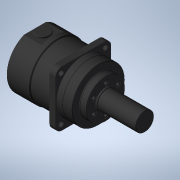
# Autodesk Inventor part: HPG-32A-33-J2NELA(400)
Saved by Autodesk Inventor 2021 (Build 250183000, 183)
## iProperties
Created: 2025-02-20
Part Number: HPG-32A-33-J2NELA(400)
Material: Generic
Catalog Web Link: www.cadenas.de
Description: HPG-32A-
Vendor: HARMONIC
Document SubType Name: Modeling
Designer: psAdmin
Manufacturer: HARMONIC
Mass: 1664.6 g
Surface Area: 1195.64 cm^2
Volume: 1664.6 cm^3
Density: 1 g/cm^3
Appearance: PSOLRGB-175-175-175
Category: PARTsolutions
Company: HARMONIC
Title: HPG-32A-33-J2NELA
Author: Cadenas PARTsolutions
PSOL_IDENT_0: {$CADENAS_DATA/23d-libs/harmonicdrive/data/hpg_series/selection_for_order_number/3d/shaft_output_no_
PSOL_IDENT_1: key_way/hpg_32a_j2.prj},182 {VTYP=3D},{NB=HPG-32A-33-J2NELA(400)},{LINA=HPG-32A-33-J2NELA},{NN=HPG-3
PSOL_IDENT_2: 2A},{DATE=16.11.2023 08:26:27},{GEOMDATE=09.08.2021 10:42:12},{VERSION=},{LINEID=4630},{WBVAR=},{WBN
PSOL_IDENT_3: UMERIC=}  {NB=HPG-32A-33-J2NELA(400)},{LINA=HPG-32A-33-J2NELA},{KT=DUMMY},{CNSORDERNO=HPG-32A-33-J2N
PSOL_IDENT_4: ELA},{R=33},{MC=400},{FN=NELA},{CNSORDERNO26=J2},{CNSORDERNO2=HPG-32A-33-J_NELA},{SB=0},{VERX=1}
NB: HPG-32A-33-J2NELA(400)
NN: HPG-32A
NBSYN: $CNSORDERNO.($MC.)
LINA: HPG-32A-33-J2NELA
CATALOG: Harmonic Drive
CNSORDERNO: HPG-32A-33-J2NELA
R: 33
MC: 400
FN: NELA
VERX: 1
SUPPLIER: HARMONIC
ARTICLENO: HPG-32A-33-J2NELA(400)
BOMINFO: HPG-32A-33-J2NELA
CREATOR: CADENAS GmbH
Autodesk Inventor part; units mm, degrees
ref_plane "YZ Plane" through (0, 0, 0) normal (1, 0, 0) x (0, 1, 0)
ref_plane "XZ Plane" through (0, 0, 0) normal (0, 1, 0) x (-1, 0, 0)
ref_plane "XY Plane" through (0, 0, 0) normal (0, 0, 1) x (1, 0, 0)
sketch "Sketch_1" plane through (0, 0, 0) normal (0, 0, 1) x (1, 0, 0)
  line L0 (237, 0) -> (38.8, 0)
  line L1 (38.8, 0) -> (38.8, 7)
  line L2 (38.8, 7) -> (12.3, 7)
  line L3 (12.3, 7) -> (11.8, 7.5)
  line L4 (11.8, 7.5) -> (11.8, 17)
  line L5 (11.8, 17) -> (12.3, 17.5)
  line L6 (12.3, 17.5) -> (27.3, 17.5)
  line L7 (27.3, 17.5) -> (27.3, 20.2)
  line L8 (27.3, 20.2) -> (27.6, 20.5)
  line L9 (27.6, 20.5) -> (30, 20.5)
  line L10 (30, 20.5) -> (30.3, 20.2)
  line L11 (30.3, 20.2) -> (30.3, 28)
  line L12 (30.3, 28) -> (10, 28)
  line L13 (10, 28) -> (10, 25)
  line L14 (10, 25) -> (0.5, 25)
  line L15 (0.5, 25) -> (0, 25.5)
  line L16 (0, 25.5) -> (0, 61)
  line L17 (0, 61) -> (48, 61)
  line L18 (48, 61) -> (50, 59)
  line L19 (50, 59) -> (104, 59)
  line L20 (104, 59) -> (104, 57.5)
  line L21 (104, 57.5) -> (116.5, 57.5)
  line L22 (116.5, 57.5) -> (117, 57)
  line L23 (117, 57) -> (136, 57)
  line L24 (136, 57) -> (137, 56)
  line L25 (137, 56) -> (137, 42)
  line L26 (137, 42) -> (138.5, 42)
  line L27 (138.5, 42) -> (139, 41.5)
  line L28 (139, 41.5) -> (139.5, 42)
  line L29 (139.5, 42) -> (151.5, 42)
  line L30 (151.5, 42) -> (152, 41.5)
  line L31 (152, 41.5) -> (152, 22)
  line L32 (152, 22) -> (155, 22)
  line L33 (155, 22) -> (155, 20.4)
  arc A0 (155, 20.4) -> (155.4, 20) centre (155.4, 20.4) ccw
  line L34 (155.4, 20) -> (236, 20)
  line L35 (236, 20) -> (237, 19)
  line L36 (237, 19) -> (237, 0)
  line L37 (237, 0) -> (38.8, 0)
  constraints: 76 end point, 2 point on circle, 1 centre point
revolve "Revolution1" add sketch "Sketch_1" angle 360 about axis through (237, 0, 0) along (1, 0, 0)
sketch "Sketch_6" plane through (0, 0, 0) normal (1, 0, 0) x (0, 1, 0)
  line L0 (0.5, 14.2) -> (-0.5, 14.2)
  line L1 (-0.5, 14.2) -> (-0.5, -17.8)
  line L2 (-0.5, -17.8) -> (0.5, -17.8)
  line L3 (0.5, -17.8) -> (0.5, 14.2)
  constraints: 8 end point
extrude "Extrusion1" cut sketch "Sketch_6" along normal blind 25.689
sketch "Sketch_2" plane through (91, 0, 0) normal (1, 0, 0) x (0, 0, -1)
  line L0 (-60, 46) -> (-60, -46)
  arc A0 (-60, -46) -> (-46, -60) centre (-46, -46) ccw
  line L1 (-46, -60) -> (46, -60)
  arc A1 (46, -60) -> (60, -46) centre (46, -46) ccw
  line L2 (60, -46) -> (60, 46)
  arc A2 (60, 46) -> (46, 60) centre (46, 46) ccw
  line L3 (46, 60) -> (-46, 60)
  arc A3 (-46, 60) -> (-60, 46) centre (-46, 46) ccw
  circle A4 centre (47.7297, -47.7297) radius 5.5
  circle A5 centre (47.7297, 47.7297) radius 5.5
  circle A6 centre (-47.7297, -47.7297) radius 5.5
  circle A7 centre (-47.7297, 47.7297) radius 5.5
  constraints: 8 centre point, 8 end point, 8 point on circle
extrude "Extrusion2" add sketch "Sketch_2" along normal blind 13
sketch "Sketch_3" plane through (16.8, 0, 0) normal (1, 0, 0) x (0, 0, -1)
  line L0 (13.5, -15) -> (13.5, 15)
  line L1 (13.5, 15) -> (17.5, 15)
  line L2 (17.5, 15) -> (17.5, 4)
  line L3 (17.5, 4) -> (15.75, 4)
  line L4 (15.75, 4) -> (15.75, -15)
  line L5 (15.75, -15) -> (13.5, -15)
  line L6 (13.5, -15) -> (13.5, 15)
  constraints: 14 end point
revolve "Revolution2" cut sketch "Sketch_3" angle 360 about axis through (16.8, -15, -13.5) along (0, -1, 0)
sketch "Sketch_4" plane through (0, 0, 0) normal (1, 0, 0) x (0, 1, 0)
  line L0 (66, 30) -> (56, 30)
  line L1 (56, 30) -> (56, -30)
  line L2 (56, -30) -> (66, -30)
  line L3 (66, -30) -> (66, 30)
  constraints: 8 end point
extrude "Extrusion3" cut sketch "Sketch_4" along normal blind 38
sketch "Sketch_5" plane through (16.8, 0, 0) normal (1, 0, 0) x (0, 0, -1)
  line L0 (13.5, -12) -> (13.5, 8)
  line L1 (13.5, 8) -> (16.7, 8)
  line L2 (16.7, 8) -> (17, 7.7)
  line L3 (17, 7.7) -> (17, 4)
  line L4 (17, 4) -> (15.75, 4)
  line L5 (15.75, 4) -> (15.75, -11.4)
  line L6 (15.75, -11.4) -> (15.15, -12)
  line L7 (15.15, -12) -> (13.5, -12)
  line L8 (13.5, -12) -> (13.5, 8)
  constraints: 18 end point
revolve "Revolution3" add sketch "Sketch_5" angle 360 about axis through (16.8, -12, -13.5) along (0, -1, 0)
sketch "Sketch7" plane through (0, 56, -24.1868) normal (0, 1, 0) x (1, 0, 0)
  point P0 (16.8, -24.1868)
hole "Hole1" at (16.8, 56, 0) direction (0, -1, 0) diameter 22 depth 33
sketch "Sketch_8" plane through (0, 8, 0) normal (0, 1, 0) x (1, 0, 0)
  line L0 (15.3, 12.634) -> (16.8, 11.7679)
  line L1 (16.8, 11.7679) -> (18.3, 12.634)
  line L2 (18.3, 12.634) -> (18.3, 14.366)
  line L3 (18.3, 14.366) -> (16.8, 15.2321)
  line L4 (16.8, 15.2321) -> (15.3, 14.366)
  line L5 (15.3, 14.366) -> (15.3, 12.634)
  constraints: 12 end point
extrude "Extrusion4" cut sketch "Sketch_8" against normal blind 2
sketch "Sketch9" plane through (0, 0, 0) normal (-1, 0, 0) x (0, 0, 1)
  point P0 (20.0909, 48.5037)
hole "Hole2" at (0, 48.5037, 20.0909) direction (1, 0, 0) diameter 9.5 depth 15
pattern_circular "Circular Pattern1" count 8 over 360 about axis through (0, 0, 0) along (1, 0, 0) of "Hole2"
sketch "Sketch_11" plane through (0, 0, 0) normal (0, -0.3826834, 0.9238795) x (1, 0, 0)
  line L0 (15, 52.5) -> (10, 52.5)
  line L1 (10, 52.5) -> (10, 56.25)
  line L2 (10, 56.25) -> (10.5, 56.75)
  line L3 (10.5, 56.75) -> (15, 56.75)
  line L4 (15, 56.75) -> (15, 52.5)
  line L5 (15, 52.5) -> (10, 52.5)
  constraints: 12 end point
revolve "Revolution4" add sketch "Sketch_11" angle 360 about axis through (15, 48.5037, 20.0909) along (1, 0, 0)
pattern_circular "Circular Pattern2" count 8 over 360 about axis through (10, 0, 0) along (1, 0, 0) of "Revolution4"
sketch "Sketch_13" plane through (10, 0, 0) normal (1, 0, 0) x (0, 0, -1)
  line L0 (-22.3805, 48.8051) -> (-21.4968, 46.6715)
  line L1 (-21.4968, 46.6715) -> (-19.2071, 46.3701)
  line L2 (-19.2071, 46.3701) -> (-17.8012, 48.2022)
  line L3 (-17.8012, 48.2022) -> (-18.685, 50.3358)
  line L4 (-18.685, 50.3358) -> (-20.9746, 50.6373)
  line L5 (-20.9746, 50.6373) -> (-22.3805, 48.8051)
  constraints: 12 end point
extrude "Extrusion5" cut sketch "Sketch_13" along normal blind 3
pattern_circular "Circular Pattern3" count 8 over 360 about axis through (10, 0, 0) along (1, 0, 0) of "Extrusion5"
sketch "Sketch12" plane through (0, 0, 0) normal (-1, 0, 0) x (0, 0, 1)
  point P0 (24.7487, 24.7487)
hole "Hole3" at (0, 24.7487, 24.7487) direction (1, 0, 0) diameter 3.242 depth 11.6 tip angle 120 countersink diameter 4 countersink angle 90 thread size "M4x0.7" class "6H" standard "ISO Metric profile"
pattern_linear "Rectangular Pattern1" count 2 spacing 49.4975 along (0, 0, -1) count 2 spacing 49.4975 along (0, -1, 0) of "Hole3"
sketch "Sketch_17" plane through (0, 0, 0) normal (0, 0, 1) x (1, 0, 0)
  line L0 (16.8, 49) -> (16.8, 59)
  line L1 (16.8, 59) -> (30.3, 59)
  arc A0 (31.8, 57.5) -> (30.3, 59) centre (30.3, 57.5) ccw
  line L2 (31.8, 57.5) -> (31.8, 56)
  line L3 (31.8, 56) -> (27.8, 56)
  line L4 (27.8, 56) -> (27.8, 49)
  line L5 (27.8, 49) -> (16.8, 49)
  line L6 (16.8, 49) -> (16.8, 59)
  constraints: 14 end point, 2 point on circle, 1 centre point
revolve "Revolution5" add sketch "Sketch_17" angle 360 about axis through (16.8, 49, 0) along (0, -1, 0)
sketch "Sketch14" plane through (152, 0, 0) normal (1, 0, 0) x (0, 0, -1)
  point P0 (0, 30)
hole "Hole4" at (152, 30, 0) direction (-1, 0, 0) diameter 14 depth 8
sketch "Sketch_20" plane through (0, 0, 0) normal (0, 0, 1) x (1, 0, 0)
  line L0 (152, 30) -> (144, 30)
  line L1 (144, 30) -> (144, 36.5)
  line L2 (144, 36.5) -> (151.5667, 36.5)
  arc A0 (152, 36.0667) -> (151.5667, 36.5) centre (151.5667, 36.0667) ccw
  line L3 (152, 36.0667) -> (152, 30)
  line L4 (152, 30) -> (144, 30)
  constraints: 10 end point, 2 point on circle, 1 centre point
revolve "Revolution6" add sketch "Sketch_20" angle 360 about axis through (152, 30, 0) along (1, 0, 0)
pattern_linear "Rectangular Pattern2" count 3 spacing 30 along (0, -0.5, 0.8660254) count 3 spacing 30 along (0, -0.5, -0.8660254) of "Hole4" skipped copies 3 5 7
pattern_linear "Rectangular Pattern3" count 3 spacing 30 along (0, -0.5, 0.8660254) count 3 spacing 30 along (0, -0.5, -0.8660254) of "Revolution6" skipped copies 3 5 7
sketch "Sketch_22" plane through (152, 0, 0) normal (1, 0, 0) x (0, 0, -1)
  line L0 (-3, 28.2679) -> (0, 26.5359)
  line L1 (0, 26.5359) -> (3, 28.2679)
  line L2 (3, 28.2679) -> (3, 31.7321)
  line L3 (3, 31.7321) -> (0, 33.4641)
  line L4 (0, 33.4641) -> (-3, 31.7321)
  line L5 (-3, 31.7321) -> (-3, 28.2679)
  constraints: 12 end point
extrude "Extrusion6" cut sketch "Sketch_22" against normal blind 4
pattern_linear "Rectangular Pattern4" count 3 spacing 30 along (0, -0.5, 0.8660254) count 3 spacing 30 along (0, -0.5, -0.8660254) of "Extrusion6" skipped copies 3 5 7
sketch "Sketch_26" plane through (22.8, 0, 0) normal (1, 0, 0) x (0, 0, -1)
  line L0 (-5, 17.2916) -> (-5, -17.2916)
  arc A0 (-5, -17.2916) -> (-5, 17.2916) centre (0, 0) ccw
  constraints: 2 end point, 2 point on circle, 1 centre point
extrude "Extrusion7" cut sketch "Sketch_26" against normal blind 1
ref_plane "IP_XY" through (0, 0, 0) normal (1, 0, 0) x (0, 0, -1)
ref_plane "IP_YZ" through (0, 0, 0) normal (0, 0, -1) x (0, 1, 0)
ref_plane "IP_ZX" through (0, 0, 0) normal (0, 1, 0) x (1, 0, 0)
body "Solid1"
